Autodesk Fusion 360 part; units mm, degrees
note: some values were not read from the file. Chosen so that the rebuilt part matches the saved one: which bodies a step acts on. Set by a fixed rule: which sketch regions a step uses.
(part 2 of 2)
  constraint parallel L180 L182
  constraint parallel L181 L183
  constraint coincident L184 P96
  constraint coincident L185 P96
  constraint coincident P96 P95
  constraint horizontal L186
  constraint perpendicular L186 L187
  constraint parallel L186 L188
  constraint parallel L187 L189
  constraint coincident L190 P96
  constraint coincident L191 P96
  constraint horizontal L628
  constraint perpendicular L309 L628
  constraint parallel L283 L628
  constraint parallel L224 L309
  constraint coincident origin L301
  constraint coincident origin L300
  constraint perpendicular L621 L636
  constraint horizontal L312
  constraint perpendicular L312 L346
  constraint parallel L270 L312
  constraint parallel L346 L352
  constraint coincident P54 L298
  constraint coincident P54 L297
  constraint symmetric P54 P59 L621
  constraint symmetric L9.start L19.start L621
  constraint symmetric L15.end L19.end L621
  constraint symmetric L14.end L20.start L621
  constraint symmetric L9.end L21.end L621
  constraint symmetric L10.start L22.start L621
  constraint symmetric L10.end L22.end L621
  constraint symmetric L23.start L11.end L621
  constraint symmetric L12.end L23.end L621
  constraint horizontal L272
  constraint perpendicular L272 L349
  constraint parallel L272 L364
  constraint parallel L335 L349
  constraint coincident P57 L319
  constraint coincident P57 L269
  constraint vertical L234
  constraint symmetric P57 P61 L234
  constraint symmetric L31.start L40.start L234
  constraint symmetric L41.start L30.end L234
  constraint symmetric L32.end L42.end L234
  constraint symmetric L40.end L29.end L234
  constraint symmetric L42.start L32.start L234
  constraint symmetric L29.start L43.end L234
  constraint symmetric L45.start L36.end L234
  constraint symmetric L33.start L44.start L234
  constraint symmetric P57 P63 L621
  constraint symmetric L31.start L55.end L621
  constraint symmetric L50.end L30.end L621
  constraint symmetric L32.end L63.end L621
  constraint symmetric L29.end L50.start L621
  constraint symmetric L32.start L60.end L621
  constraint symmetric L51.start L29.start L621
  constraint symmetric L36.end L56.start L621
  constraint symmetric L56.end L33.start L621
  constraint symmetric L41.start L54.end L621
  constraint symmetric L44.start L52.end L621
  constraint symmetric L40.start L57.start L621
  constraint symmetric P61 P64 L621
  constraint symmetric L42.start L61.start L621
  constraint symmetric L45.start L52.start L621
  constraint symmetric L53.start L43.end L621
  constraint symmetric L42.end L58.start L621
  constraint symmetric L53.end L40.end L621
  constraint symmetric P64 P61 L621
  constraint coincident P66 L311
  constraint coincident P66 L316
  constraint perpendicular L271 L277
  constraint symmetric P66 P70 L277
  constraint symmetric L72.start L80.start L277
  constraint symmetric L74.end L78.end L277
  constraint symmetric L71.start L81.start L277
  constraint symmetric L72.end L80.end L277
  constraint symmetric L73.start L77.end L277
  constraint symmetric L74.start L78.start L277
  constraint symmetric L70.start L79.start L277
  constraint symmetric L70.end L77.start L277
  constraint symmetric P66 P71 L234
  constraint symmetric L72.start L84.start L234
  constraint symmetric L74.end L83.end L234
  constraint symmetric L71.start L87.end L234
  constraint symmetric L72.end L84.end L234
  constraint symmetric L73.start L87.start L234
  constraint symmetric L74.start L83.start L234
  constraint symmetric L70.start L86.start L234
  constraint symmetric L70.end L86.end L234
  constraint symmetric L76.start L95.start L234
  constraint symmetric L76.end L95.end L234
  constraint symmetric L78.end L94.end L234
  constraint symmetric P70 P72 L234
  constraint symmetric L89.start L77.start L234
  constraint symmetric L81.start L85.start L234
  constraint symmetric L79.start L85.end L234
  constraint symmetric L94.start L78.start L234
  constraint symmetric P72 P70 L234
  constraint symmetric L93.end L80.end L234
  constraint symmetric L89.end L77.end L234
  constraint symmetric L80.start L93.start L234
  constraint symmetric P47 L39.end L621
  constraint symmetric P44 P66 L621
  constraint symmetric L103.start L72.start L621
  constraint symmetric L109.end L74.end L621
  constraint symmetric L107.start L71.start L621
  constraint symmetric L103.end L72.end L621
  constraint symmetric L112.end L73.start L621
  constraint symmetric L109.start L74.start L621
  constraint symmetric L107.end L70.start L621
  constraint symmetric L70.end L110.end L621
  constraint symmetric L111.end L78.end L621
  constraint symmetric P45 P70 L621
  constraint symmetric L105.end L77.start L621
  constraint symmetric L96.end L81.start L621
  constraint symmetric L105.start L79.start L621
  constraint symmetric L111.start L78.start L621
  constraint symmetric L108.end L80.end L621
  constraint symmetric L96.start L77.end L621
  constraint symmetric L108.start L80.start L621
  constraint symmetric L115.end L84.end L621
  constraint symmetric L99.end L86.end L621
  constraint symmetric L98.end L85.start L621
  constraint symmetric L102.start L93.start L621
  constraint symmetric P46 P71 L621
  constraint symmetric L115.start L84.start L621
  constraint symmetric P43 P72 L621
  constraint symmetric L104.end L94.end L621
  constraint symmetric L114.start L83.start L621
  constraint symmetric L98.start L89.end L621
  constraint symmetric L87.start L106.end L621
  constraint symmetric L97.end L89.start L621
  constraint symmetric L117.end L87.end L621
  constraint symmetric L97.start L85.end L621
  constraint symmetric L94.start L104.start L621
  constraint symmetric L93.end L102.end L621
  constraint symmetric L99.start L86.start L621
  constraint symmetric L114.end L83.end L621
  constraint midpoint L120.start L221
  constraint parallel L213 L221
  constraint parallel L192 L221
  constraint parallel L216 L222
  constraint midpoint L125.start L278
  constraint perpendicular L246 L382
  constraint perpendicular L246 L376
  constraint midpoint P48 L355
  constraint midpoint L127.start L265
  constraint midpoint P39 L289
  constraint coincident L129.end L289
  constraint parallel L264 L273
  constraint symmetric L125.end L131.start L234
  constraint symmetric L126.end L130.start L234
  constraint symmetric L129.end L131.end L234
  constraint symmetric L125.end L133.start L621
  constraint symmetric L126.end L132.start L621
  constraint symmetric L129.end L133.end L621
  constraint symmetric L130.start L134.start L621
  constraint symmetric L131.start L135.start L621
  constraint symmetric L131.end L135.end L621
  constraint midpoint P49 L330
  constraint midpoint P50 L365
  constraint midpoint L136.start L357
  constraint midpoint P51 L279
  constraint midpoint P52 L274
  constraint parallel L330 L336
  constraint parallel L306 L330
  constraint coincident L140.end L357
  constraint coincident L141.end L279
  constraint parallel L337 L338
  constraint symmetric L138.end L143.start L277
  constraint symmetric L143.end L140.end L277
  constraint symmetric L141.end L142.end L277
  constraint symmetric L138.end L147.start L234
  constraint symmetric L140.end L147.end L234
  constraint symmetric L146.end L141.end L234
  constraint symmetric L145.end L142.end L234
  constraint symmetric L144.start L143.start L234
  constraint symmetric L143.end L144.end L234
  constraint symmetric L138.end L151.start L621
  constraint symmetric L140.end L151.end L621
  constraint symmetric L141.end L150.end L621
  constraint symmetric L142.end L149.end L621
  constraint symmetric L143.start L148.start L621
  constraint symmetric L143.end L148.end L621
  constraint symmetric L144.start L155.start L621
  constraint symmetric L144.end L155.end L621
  constraint symmetric L145.end L154.end L621
  constraint symmetric L146.end L153.end L621
  constraint symmetric L147.start L152.start L621
  constraint symmetric L152.end L147.end L621
  constraint perpendicular L267 L356
  constraint coincident L621.start L331
  constraint coincident L621.start L194
  constraint tangent L331 A15
  constraint tangent L194 A15
  constraint tangent L331 A8
  constraint tangent A8 L356
  constraint tangent L194 A6
  constraint tangent A6 L304
  constraint tangent L356 A9
  constraint tangent L267 A9
  constraint tangent L267 A7
  constraint tangent A7 L304
  constraint coincident L170.start L356
  constraint coincident P96 L621
  constraint symmetric L159.start L163.start L621
  constraint symmetric L161.end L162.end L621
  constraint symmetric L159.end L163.end L621
  constraint symmetric L160.start L164.start L621
  constraint symmetric L161.start L162.start L621
  constraint midpoint L167.end L267
  constraint coincident L165.start L621
  constraint coincident L165.end A5
  constraint coincident L165.end L621
  constraint collinear L236 L243
  constraint parallel L218 L371
  constraint coincident L172.start L304
  constraint collinear L286 L304
  constraint coincident L173.start L286
  constraint collinear L286 L299
  constraint horizontal L632
  constraint perpendicular L320 L632
  constraint parallel L313 L632
  constraint parallel L223 L320
  constraint horizontal L215
  constraint perpendicular L215 L351
  constraint parallel L215 L268
  constraint parallel L201 L351
  constraint coincident P96 L205
  constraint coincident P96 L200
  constraint horizontal L203
  constraint perpendicular L203 L322
  constraint parallel L203 L317
  constraint parallel L198 L322
  constraint coincident P96 L197
  constraint coincident P96 L195
  constraint horizontal L395
  constraint perpendicular L387 L395
  constraint parallel L388 L395
  constraint parallel L387 L408
  constraint coincident P75 L401
  constraint coincident P75 L393
  constraint coincident P75 P74
  constraint horizontal L396
  constraint perpendicular L386 L396
  constraint parallel L389 L396
  constraint parallel L386 L409
  constraint coincident P75 L397
  constraint coincident P75 L390
  constraint perpendicular L394 L396
  constraint coincident L404.end A13
  constraint midpoint L405.end L386
  constraint parallel L405 L407
  constraint coincident L407.end L386
  constraint coincident L406.end A13
  constraint parallel L404 L406
  constraint symmetric L404.start L385.start L394
  constraint symmetric L404.end L385.end L394
  constraint symmetric L405.end L391.end L394
  constraint symmetric L407.end L398.end L394
  constraint symmetric L406.start L402.start L394
  constraint symmetric L406.end L403.end L394
  constraint concentric A12 A13
  constraint coincident L391.start A10
  constraint coincident L398.start A10
  constraint coincident A17.start A16
  constraint concentric A15 A19
  constraint concentric A16 A17
  constraint symmetric A17.start L411.end L621
  constraint symmetric A15.end L410.end L621
  constraint coincident L411 A17.end
  constraint concentric A17 A18
  constraint concentric A19 A20
  constraint coincident L410 A18.start
  constraint coincident A21 L412.end
  constraint parallel L159 L412
  constraint horizontal L430
  constraint perpendicular L419 L430
  constraint parallel L430 L432
  constraint parallel L419 L427
  constraint coincident P96 L416
  constraint coincident P96 L421
  constraint horizontal L434
  constraint perpendicular L414 L434
  constraint parallel L434 L435
  constraint parallel L413 L414
  constraint coincident P96 L424
  constraint coincident P96 L415
  constraint horizontal L431
  constraint perpendicular L422 L431
  constraint parallel L428 L431
  constraint parallel L422 L429
  constraint coincident P96 L420
  constraint coincident P96 L425
  constraint horizontal L433
  constraint perpendicular L418 L433
  constraint parallel L433 L436
  constraint parallel L418 L423
  constraint coincident P96 L426
  constraint coincident P96 L417
  constraint horizontal L454
  constraint perpendicular L443 L454
  constraint parallel L454 L456
  constraint parallel L443 L451
  constraint coincident P96 L440
  constraint coincident P96 L445
  constraint horizontal L458
  constraint perpendicular L438 L458
  constraint parallel L458 L459
  constraint parallel L437 L438
  constraint coincident P96 L448
  constraint coincident P96 L439
  constraint horizontal L455
  constraint perpendicular L446 L455
  constraint parallel L452 L455
  constraint parallel L446 L453
  constraint coincident P96 L444
  constraint coincident P96 L449
  constraint horizontal L457
  constraint perpendicular L442 L457
  constraint parallel L457 L460
  constraint parallel L442 L447
  constraint coincident P96 L450
  constraint coincident P96 L441
  constraint horizontal L478
  constraint perpendicular L467 L478
  constraint parallel L478 L480
  constraint parallel L467 L475
  constraint coincident P96 L464
  constraint coincident P96 L469
  constraint horizontal L482
  constraint perpendicular L462 L482
  constraint parallel L482 L483
  constraint parallel L461 L462
  constraint coincident P96 L472
  constraint coincident P96 L463
  constraint horizontal L479
  constraint perpendicular L470 L479
  constraint parallel L476 L479
  constraint parallel L470 L477
  constraint coincident P96 L468
  constraint coincident P96 L473
  constraint horizontal L481
  constraint perpendicular L466 L481
  constraint parallel L481 L484
  constraint parallel L466 L471
  constraint coincident P96 L474
  constraint coincident P96 L465
  constraint coincident A21 L493.end
  constraint parallel L199 L493
  constraint coincident A21 L494.end
  constraint perpendicular L496 L497
  constraint parallel L496 L500
  constraint perpendicular L514 L515
  constraint parallel L513 L515
  constraint parallel L514 L517
  constraint symmetric L39 L513.end L520.start
  constraint symmetric L39 L515.start L520.end
  constraint symmetric L39 L511.start L521.end
  constraint symmetric L39 L511.end L524.end
  constraint symmetric L39 L513.start L523.end
  constraint symmetric L39 L514.start L522.end
  constraint symmetric L39 L516.start L519.end
  constraint symmetric L39 L512.end L519.start
  constraint symmetric L277 L543.end L547.end
  constraint symmetric L277 L543.start L547.start
  constraint symmetric L277 L545.end L549.start
  constraint symmetric L277 L544.start L548.start
  constraint symmetric L39 L543.end L551.end
  constraint symmetric L39 L543.start L551.start
  constraint symmetric L39 L545.end L553.start
  constraint symmetric L39 L544.start L552.start
  constraint symmetric L39 L547.start L555.start
  constraint symmetric L39 L547.end L555.end
  constraint symmetric L39 L548.start L556.start
  constraint symmetric L39 L549.start L557.end
  constraint coincident L508 L123.start
  constraint coincident L508 L122.start
  constraint coincident L498 L124.start
  constraint coincident L498 L307.start
  constraint coincident L485 L124.end
  constraint coincident L485 L307.end
  constraint coincident L486 L123.end
  constraint coincident L486 L122.end
  constraint coincident L492 L405.start
  constraint coincident L499 L128.end
  constraint coincident L501 L130.end
  constraint coincident L543 L142.start
  constraint coincident L547 L141.start
  constraint coincident L555 L146.start
  constraint coincident L551 L145.start
  constraint coincident L573 L154.start
  constraint coincident L569 L153.start
  constraint coincident L566 L150.start
  constraint coincident L560 L149.start
  constraint perpendicular L577 L581
  constraint parallel L577 L582
  constraint parallel L578 L581
  constraint perpendicular L580 L583
  constraint parallel L576 L583
  constraint parallel L579 L580
  constraint coincident A13 A22.start
  constraint coincident A12 A22.end
  constraint symmetric L394 A13.start A13.end
  constraint symmetric L394 A22.start A25.end
  constraint symmetric L394 A22 A25
  constraint symmetric L394 A23 A24
  constraint symmetric L394 A22.end A25.start
  constraint symmetric L394 A12.end A12.start
  constraint tangent A15 S0
  constraint tangent A19 S1
  constraint concentric A30 A31
  constraint coincident A31.end S0
  constraint coincident A31.start S1
  constraint midpoint A30.end L584
  constraint midpoint A30.start L585
  constraint tangent A19 S2
  constraint tangent A18 S3
  constraint coincident A32 S2.end
  constraint midpoint S2.end L588
  constraint coincident A32 S3.start
  constraint midpoint S3.start L589
  constraint coincident A32 L586.end
  constraint coincident A32 L587.end
  constraint concentric A33 A34
  constraint concentric A35 A36
  constraint coincident A34.start S5
  constraint coincident A34.end S6
  constraint coincident A35.end S6
  constraint coincident A35.start S4
  constraint midpoint A36.start L590
  constraint midpoint A33.start L591
  constraint midpoint A33.end L592
  constraint midpoint A36.end L593
  constraint midpoint A37.end L594
  constraint collinear L595 L596
  constraint midpoint A37.start L597
  constraint midpoint A39.start L598
  constraint midpoint A39.end L599
  constraint concentric A41 A42
  constraint coincident A41.end L600
  constraint coincident A41.start L600
  constraint coincident A42.end L600
  constraint collinear L600 L601
  constraint symmetric L234 A41.end A43.start
  constraint symmetric L234 A41.start A43.end
  constraint symmetric L234 A41 A43
  constraint symmetric L234 A42.end A44.start
  constraint symmetric L234 A42.start A44.end
  constraint symmetric L234 A42 A44
  constraint concentric A45 A46
  constraint coincident A46.start L601
  constraint coincident A45.start L601
  constraint coincident A46.end L601
  constraint collinear L601 L602
  constraint collinear L602 L603
  constraint coincident L286 L605.end
  constraint perpendicular L286 L604
  constraint collinear L604 L606
  constraint collinear L605 L606
  constraint collinear L606 L607
  constraint symmetric A52.start L606 L606.start
  constraint symmetric L604.end L606 A52.end
  constraint symmetric A49.start L606 L606.end
  constraint symmetric L607.start L606 A49.end
  constraint symmetric L605.start L606 A47.start
  constraint symmetric L607.end L606 A47.end
  constraint coincident A53 S10.end
  constraint midpoint S10.end L608
  constraint coincident A53 S11.start
  constraint midpoint S11.start L609
  constraint coincident A54 S12.end
  constraint midpoint S12.end L610
  constraint coincident A54 S13.start
  constraint midpoint S13.start L611
  constraint coincident S11 A55.end
  constraint coincident S10 A56.start
  constraint concentric A55 A56
  constraint tangent A2 L612
  constraint collinear L612 L613
  constraint coincident A58 L613.end
  constraint coincident A58 L614.start
  constraint collinear L613 L614
  constraint parallel L167 L619
  constraint symmetric L39 A58 A59
  constraint tangent A60 L615
  constraint tangent A60 L616
  constraint collinear L618 L621
  constraint coincident L615 L619.end
  constraint coincident L616 L620.start
  constraint collinear L619 L620
  constraint concentric A59 A60
  constraint coincident A65 L621.end
  constraint coincident A65 L624.start
  constraint collinear L621 L624
  constraint coincident A65 L622.end
  constraint coincident A65 L623.start
  constraint collinear L622 L623
  constraint coincident A61 L624.end
  constraint coincident A61 L625.start
  constraint collinear L624 L625
  constraint coincident A61 L166.start
  constraint coincident A61 L623.end
  constraint coincident L491 L626.end
  constraint collinear L626 L627
  constraint coincident L489 L627.start
  constraint collinear L628 L629
  constraint collinear L630 L631
  constraint collinear L632 L633
  constraint coincident L491 L634.end
  constraint coincident L621 L635.start
  constraint collinear L634 L635
  constraint collinear L636 L637
  constraint tangent A58 S14
  constraint tangent A58 S15
  measures "d1" distance of L0.end L1.end
  measures "d2" distance of L0.start L0.end
  measures "d4" distance of L6.end L7.end
  measures "d6" distance of L15.end L9.end
  measures "d7" distance of L9.start L15.end
  measures "d8" distance of L10.start L12.end
  measures "d10" distance of L30.end L29.end
  measures "d11" distance of L29.end L29.start
  measures "d12" distance of L32.end L32.start
  measures "d14" distance of L74.end L72.end
  measures "d15" distance of L72.end L74.start
  measures "d16" distance of L71.start L73.start
  measures "d20" distance of L120.start L120.end
  measures "d21" distance of L120.start L121.end
  measures "d22" angle of L26 L122
  measures "d23" distance of L125.start L125.end L44.start
  measures "d24" distance of L125.start L126.end L44.start
  measures "d27" distance of P49 L138.end
  measures "d28" distance of P49 L139.end
  measures "d30" distance of L86 L156
  measures "d31" radius of A16
  measures "d32" radius of A0
  measures "d34" radius of A2
  measures "d36" diameter of A4
  measures "d90" distance of L0.end L1.end
  measures "d91" distance of L0.start L0.end
  measures "d92" distance of L7.end L6.end
  measures "d93" distance of L181.end L182.end
  measures "d94" distance of L180.end L181.end
  measures "d95" distance of L187.end L188.end
  measures "d96" distance of L186.end L187.end
  measures "d107" distance of L0.end L1.end
  measures "d108" distance of L0.start L0.end
  measures "d109" distance of L7.end L6.end
  measures "d110" distance of L15.end L9.end
  measures "d111" distance of L9.start L15.end
  measures "d112" distance of L10.start L12.end
  measures "d113" distance of L30.end L29.end
  measures "d114" distance of L29.start L29.end
  measures "d115" distance of L32.end L32.start
  measures "d116" distance of L74.end L72.end
  measures "d117" distance of L72.end L74.start
  measures "d118" distance of L71.start L73.start
  measures "d119" distance of L120.start L120.end
  measures "d120" distance of L120.start L121.end
  measures "d121" angle of L221 L222
  measures "d122" distance of L125.end L125.start
  measures "d123" distance of L126.end L125.start
  measures "d124" distance of L138.end P49
  measures "d125" distance of P49 L139.end
  measures "d126" distance of L267 L360
  measures "d127" radius of A15
  measures "d128" radius of A8
  measures "d129" radius of A9
  measures "d130" diameter of A5
  measures "d147" distance of L1.end L0.end
  measures "d148" distance of L0.start L0.end
  measures "d149" distance of L7.end L6.end
  measures "d150" distance of L182.end L181.end
  measures "d151" distance of L180.end L181.end
  measures "d152" distance of L187.end L188.end
  measures "d153" distance of L187.end L186.end
  measures "d164" diameter of A13
  measures "d165" distance of L387.end L388.end
  measures "d166" distance of L387.end L387.start
  measures "d167" distance of L389.end L386.end
  measures "d168" distance of L386.end L386.start
  measures "d191" distance of L182.end L181.end
  measures "d192" distance of L181.end L180.end
  measures "d193" distance of L188.end L187.end
  measures "d194" distance of L186.end L187.end
  measures "d195" distance of L181.end L182.end
  measures "d196" distance of L181.end L180.end
  measures "d197" distance of L187.end L188.end
  measures "d198" distance of L187.end L186.end
  measures "d199" distance of L182.end L181.end
  measures "d200" distance of L181.end L180.end
  measures "d201" distance of L188.end L187.end
  measures "d202" distance of L186.end L187.end
  measures "d203" distance of L181.end L182.end
  measures "d204" distance of L181.end L180.end
  measures "d205" distance of L187.end L188.end
  measures "d206" distance of L187.end L186.end
  measures "d207" distance of L182.end L181.end
  measures "d208" distance of L181.end L180.end
  measures "d209" distance of L188.end L187.end
  measures "d210" distance of L186.end L187.end
  measures "d211" distance of L181.end L182.end
  measures "d212" distance of L181.end L180.end
  measures "d213" distance of L187.end L188.end
  measures "d214" distance of L187.end L186.end
  measures "d215" distance of L489.start L488.start
  measures "d216" distance of L490.start L486.end
  measures "d217" distance of L487.start L488.start
  measures "d218" distance of L500.start L496.end
  measures "d219" distance of L496.end L496.start
  measures "d220" distance of L498.start L495.start
  measures "d221" distance of L496.end L500.start
  measures "d222" distance of L513.end L513.start
  measures "d223" distance of L513.start L514.start
  measures "d224" distance of L511.start L516.start
  measures "d226" distance of L543.end L543.start
  measures "d300" distance of L578.start L581.end
  measures "d301" distance of L581.end L577.end
  measures "d302" distance of L576.start L576.end
  measures "d303" distance of L576.start L580.start
  measures "d376" radius of A58
  measures "d377" radius of A57
extrude "Extrusão73" add sketch "Esboço1" along normal blind 4 contours L7 L8 L158 L161 L179 L266 L307 L314 L315 L321 L331 A18 A20 L485 L490 L559 A32 L587 S3 L589 A33 S5 L591 S6 L592 L635 L637 | L405 A17 A19 L490 L492 A31 S1 A32 L586 S2 | L5 L8 L124 A4 L159 L160 L174 L179 A5 L214 L233 L308 L314 L318 L321 L345 L485 A35 S4 S6 L593 | L5 L6 L122 A4 L163 L164 L174 L175 A5 L199 L214 L217 L222 L225 L228 L233 L486 A38 S7 S8 L597 | L6 L7 L123 L157 L162 L175 L194 L216 L225 L227 L228 L266 L407 A15 A16 L486 L492 A31 S0 A39 S8 L598 S9 L599 L634 L636 makes body 1 at (50.6885, -2.7666, 4) makes body 2 at (-4.4582, 27.7889, 4) makes body 3 at (41.1604, -31.7588, 0) makes body 4 at (-50.6869, -2.7681, 0) makes body 5 at (-41.1604, -31.7588, 0)
extrude "Extrusão74" add sketch "Esboço1" along normal blind 2 contours L0 L178 L309 L320 L490 L627 L629 L631 L633 | L0 L7 L8 L178 L179 L266 L309 L314 L320 L321 L490 L627 L629 L631 L633 L635 L637 | L0 L178 L309 L320 L489 L490 L627 L629 L631 L633 | L0 L8 L178 L179 L309 L314 L320 L321 L489 L490 | L7 L266 L489 L490 L627 L629 L631 L633 L635 L637 | L0 L1 L2 L7 L176 L177 L178 L223 L224 L266 L283 L309 L313 L320 L487 L488 L489 L491 L635 L637 | L0 L8 L178 L179 L309 L314 L320 L321 L488 L489 | L8 L179 L314 L321 L485 L488 L489 L490 | L7 L266 L489 L490 L491 L492 L634 L635 L636 L637 | L0 L1 L177 L178 L283 L309 L313 L320 L485 L488 | L0 L8 L178 L179 L309 L314 L320 L321 L485 L488 | L8 L179 L314 L321 L488 L489 | L7 L266 L489 L491 L635 L637 | L0 L1 L177 L178 L283 L309 L313 L320 L485 | L0 L1 L5 L8 L174 L177 L178 L179 L214 L233 L283 L309 L313 L314 L320 L321 L485 | L1 L5 L174 L177 L214 L233 L283 L313 L485 L488 | L1 L5 L174 L177 L214 L233 L283 L313 L487 L488 | L1 L2 L176 L177 L223 L224 L283 L313 L486 L487 | L1 L5 L174 L177 L214 L233 L283 L313 L486 L487 | L5 A4 L174 A5 L214 L233 L485 L486 L487 L488 | L5 L174 L214 L233 L487 L488 | L7 L266 L491 L492 L626 L628 L630 L632 L634 L636 | L1 L2 L176 L177 L223 L224 L283 L313 L486 | L1 L2 L5 L6 L174 L175 L176 L177 L214 L223 L224 L225 L228 L233 L283 L313 L486 | L2 L6 L175 L176 L223 L224 L225 L228 L486 L487 | L2 L6 L175 L176 L223 L224 L225 L228 L487 L491 | L2 L6 L7 L175 L176 L223 L224 L225 L228 L266 L492 L626 L628 L630 L632 L634 L636 | L2 L176 L223 L224 L491 L492 L626 L628 L630 L632 | A4 A5 A21 L412 L485 L486 L493 | L2 L6 L175 L176 L223 L224 L225 L228 L491 L492 | L6 L175 L225 L228 L486 L487 L491 L492 | L6 L175 L225 L228 L487 L491 | L2 L176 L223 L224 L492 L626 L628 L630 L632 bodies 1 5 2 3 4
extrude "Extrusão75" add sketch "Esboço1" along normal blind 6 contours L7 L266 L490 A32 L586 L587 L635 L637 | L124 L307 L308 L485 L559 S6 | L7 L266 L405 L407 L492 A31 L634 L636 | L122 L123 L216 L222 L486 S8 bodies 1
extrude "Extrusão76" add sketch "Esboço1" along normal blind 4 separate body contours L10 L11 L13 L32 L36 L37 L131 L143 L158 A0 L161 L170 L171 L265 L271 L281 L307 L310 L315 L323 L329 L331 L339 A8 L350 L356 L357 L495 L498 L501 L511 L512 L516 L559 A34 S5 S6 L592 A42 L600 L601 A57 L612 L613 | L11 L12 L13 L42 L45 L47 L124 L129 L144 A4 L159 L160 L165 L166 A5 L229 L243 L264 L265 L278 L308 L310 L318 L340 L344 L345 L354 L355 L498 L499 L521 L524 L525 A36 S4 L590 S6 L593 A44 L602 L603 L604 A62 A64 A65 L622 L623 | L32 L33 L37 L42 L44 L45 L128 L130 L140 L147 L271 L273 L278 L280 L334 L338 L340 L342 L353 L357 L499 L501 L516 L518 L519 L521 A46 L601 L602 | L145 L146 L325 L348 L519 L525 L602 | L141 L142 L333 L337 L512 L518 L601 makes body 6 at (-61.0053, -127.9109, 0) makes body 7 at (-100, -146.0948, 0) makes body 8 at (-148.8162, -124.6972, 0) makes body 9 at (-150, -213.7, 0) makes body 10 at (-50, -213.7, 0)
extrude "Extrusão77" add sketch "Esboço1" along normal blind 6 contours L124 L307 L308 L498 L559 S6 | L11 L128 L129 L264 L265 L273 L499 L521 | L11 L130 L131 L265 L280 L281 L501 L516 | L45 L144 L145 L340 L348 L354 L525 L602 | L37 L142 L143 L333 L350 L357 L512 L601 | L45 L146 L147 L325 L340 L353 L519 L602 | L37 L140 L141 L337 L338 L357 L518 L601 bodies 6 7 8
extrude "Extrusão78" add sketch "Esboço1" along normal blind 2 contours L13 L310 L495 L496 L497 L498 | A4 A5 A21 L412 L494 | L13 L17 L310 L312 L497 L498 | L12 L13 L14 L17 L310 L312 L352 L355 L498 | L10 L13 L17 L18 L310 L312 L329 L346 L495 | L13 L17 L310 L312 L495 L496 | L13 L17 L310 L312 L496 L497 | L13 L310 L496 L497 | L14 L17 L312 L352 L497 L498 | L14 L17 L312 L352 L498 | L17 L18 L312 L346 L495 | L17 L18 L312 L346 L495 L496 | L12 L355 L497 L498 L499 L500 | L12 L14 L352 L355 L497 L498 | L14 L16 L17 L18 L270 L312 L346 L352 L496 L497 L500 L502 | L10 L18 L329 L346 L495 L496 | L10 L329 L495 L496 L501 L502 | L12 L355 L497 L500 | L12 L14 L352 L355 L497 L500 | L10 L18 L329 L346 L496 L502 | L10 L329 L496 L502 | L12 L14 L352 L355 L499 L500 | L11 L12 L14 L16 L265 L270 L352 L355 L499 | L14 L16 L270 L352 L499 L500 | L16 L18 L270 L346 L501 L502 | L10 L18 L329 L346 L501 L502 | L10 L11 L16 L18 L265 L270 L329 L346 L501 | L14 L16 L270 L352 L499 | L11 L16 L265 L270 L500 L502 | L11 L16 L265 L270 L499 L500 | L16 L18 L270 L346 L501 | L11 L16 L265 L270 L501 L502 | L11 L265 L500 L502 | L11 L265 L499 L500 L501 L502 | L42 L129 L264 L278 L521 L522 L523 L524 | L128 L129 L264 L273 L521 L522 | L130 L131 L280 L281 L515 L516 | L32 L131 L271 L281 L511 L514 L515 L516 | L42 L129 L264 L278 L522 L523 | L42 L128 L129 L264 L273 L278 L522 | L42 L128 L273 L278 L521 L522 | L32 L130 L131 L271 L280 L281 L515 | L32 L131 L271 L281 L514 L515 | L32 L130 L271 L280 L515 L516 | L42 L43 L278 L282 L522 L523 | L42 L128 L273 L278 L522 | L41 L42 L43 L44 L278 L282 L327 L334 L521 | L42 L43 L278 L282 L521 L522 | L42 L43 L278 L282 L523 L524 | L42 L43 L47 L49 L278 L282 L343 L344 L524 | L32 L38 L271 L272 L514 L515 | L32 L130 L271 L280 L515 | L32 L38 L271 L272 L515 L516 | L32 L33 L34 L38 L271 L272 L335 L342 L516 | L29 L32 L36 L38 L271 L272 L323 L349 L511 | L32 L38 L271 L272 L511 L514 | L41 L43 L282 L327 L521 | L41 L43 L282 L327 L521 L522 | L43 L49 L282 L343 L523 L524 | L43 L49 L282 L343 L524 | L34 L38 L272 L335 L515 L516 | L34 L38 L272 L335 L516 | L29 L38 L272 L349 L511 | L29 L38 L272 L349 L511 L514 | L41 L43 L46 L49 L282 L324 L327 L343 L520 L522 L523 L526 | L41 L44 L327 L334 L521 L522 | L44 L334 L519 L520 L521 L522 | L47 L344 L523 L524 L525 L526 | L47 L49 L343 L344 L523 L524 | L29 L30 L34 L38 L272 L335 L349 L364 L513 L514 L515 L517 | L33 L342 L515 L516 L517 L518 | L33 L34 L335 L342 L515 L516 | L29 L36 L323 L349 L511 L514 | L36 L323 L511 L512 L513 L514 | L45 L46 L47 L49 L324 L340 L343 L344 L525 | L47 L49 L343 L344 L523 L526 | L41 L44 L327 L334 L520 L522 | L44 L334 L520 L522 | L47 L344 L523 L526 | L29 L36 L323 L349 L513 L514 | L33 L34 L335 L342 L515 L517 | L33 L342 L515 L517 | L36 L323 L513 L514 | L29 L30 L36 L37 L323 L349 L357 L364 L512 | L45 L46 L324 L340 L525 L526 | L45 L145 L146 L325 L340 L348 L519 L520 L525 L526 | L47 L49 L343 L344 L525 L526 | L46 L49 L324 L343 L525 L526 | L41 L46 L324 L327 L519 L520 | L41 L44 L327 L334 L519 L520 | L41 L44 L45 L46 L324 L327 L334 L340 L519 | L29 L30 L349 L364 L512 L513 | L29 L36 L323 L349 L512 L513 | L33 L34 L335 L342 L517 L518 | L30 L34 L335 L364 L517 L518 | L30 L33 L34 L37 L335 L342 L357 L364 L518 | L30 L37 L357 L364 L512 L513 | L37 L142 L333 L357 L512 | L37 L141 L142 L333 L337 L357 L512 L513 L517 L518 | L46 L49 L324 L343 L525 | L45 L46 L324 L340 L520 L526 | L41 L46 L324 L327 L519 | L45 L46 L324 L340 L519 L520 | L29 L30 L349 L364 L512 | L30 L37 L357 L364 L513 L517 | L30 L34 L335 L364 L518 | L30 L37 L357 L364 L517 L518 | L37 L141 L337 L357 L518 | L45 L340 L520 L526 | L37 L357 L513 L517 bodies 6 9 10
extrude "Extrusão79" add sketch "Esboço1" along normal blind 4 separate body contours L23 L24 L26 L52 L58 L61 L122 L133 L155 A4 L163 L164 L165 L166 A5 L196 L199 L208 L217 L219 L220 L221 L222 L229 L243 L245 L251 L255 L506 L508 L537 L540 L542 A37 S7 L594 S8 L597 L604 L606 A51 A61 A63 A66 L622 L623 | L22 L24 L26 L56 L63 L65 L123 L135 L148 L157 A1 L162 L172 L173 L194 L202 L207 L209 L216 L220 L221 L227 A6 L258 L286 L293 L299 L303 L504 L508 L510 L527 L530 L534 A40 S8 L598 S9 L605 L607 A48 A53 S10 L608 S11 L609 | L153 L154 L252 L253 L535 L542 L606 | L52 L56 L60 L61 L63 L67 L132 L134 L151 L152 L206 L209 L210 L219 L245 L248 L260 L263 L293 L302 L504 L506 L532 L534 L535 L537 L606 L607 A49 | L149 L150 L284 L285 L530 L532 L607 makes body 11 at (148.8208, -124.6973, 0) makes body 12 at (100, -146.0948, 0) makes body 13 at (150, -213.7, 0) makes body 14 at (61.0053, -127.9109, 0) makes body 15 at (50, -213.7, 0)
extrude "Extrusão80" add sketch "Esboço1" along normal blind 6 contours L122 L123 L216 L222 L508 S8 | L52 L154 L155 L245 L251 L253 L542 L606 | L24 L132 L133 L208 L210 L220 L506 L537 | L52 L152 L153 L245 L248 L252 L535 L606 | L24 L134 L135 L206 L207 L220 L504 L534 | L56 L150 L151 L285 L293 L302 L532 L607 | L56 L148 L149 L284 L293 L303 L530 L607 bodies 11 12 13 14 15
extrude "Extrusão81" add sketch "Esboço1" along normal blind 2 contours A4 A5 A21 L493 L494 | L26 L221 L507 L508 L509 L510 | L20 L23 L25 L26 L196 L204 L221 L232 L508 | L20 L26 L221 L232 L507 L508 | L26 L221 L507 L509 | L20 L26 L221 L232 L507 L509 | L20 L25 L204 L232 L508 | L20 L25 L204 L232 L507 L508 | L20 L26 L221 L232 L509 L510 | L19 L20 L22 L26 L193 L202 L221 L232 L510 | L23 L25 L196 L204 L507 L508 | L23 L196 L505 L506 L507 L508 | L19 L20 L25 L27 L193 L204 L212 L232 L503 L505 L507 L509 | L19 L20 L193 L232 L509 L510 | L19 L20 L193 L232 L510 | L23 L25 L196 L204 L505 L507 | L23 L196 L505 L507 | L22 L202 L503 L504 L509 L510 | L19 L22 L193 L202 L509 L510 | L23 L25 L196 L204 L505 L506 | L23 L24 L25 L27 L196 L204 L212 L220 L506 | L19 L22 L193 L202 L503 L509 | L25 L27 L204 L212 L505 L506 | L22 L202 L503 L509 | L25 L27 L204 L212 L506 | L19 L22 L193 L202 L503 L504 | L19 L27 L193 L212 L503 L504 | L24 L27 L212 L220 L505 L506 | L24 L27 L212 L220 L503 L505 | L19 L22 L24 L27 L193 L202 L212 L220 L504 | L19 L27 L193 L212 L504 | L24 L27 L212 L220 L503 L504 | L24 L132 L134 L206 L210 L220 L503 L504 L505 L506 | L24 L220 L503 L505 | L52 L53 L58 L69 L245 L255 L256 L384 L542 | L24 L132 L210 L220 L506 | L132 L133 L208 L210 L537 L538 | L61 L133 L208 L219 L537 L538 L539 L540 | L52 L69 L245 L384 L541 L542 | L52 L154 L245 L253 L542 | L52 L153 L154 L245 L252 L253 L535 L536 L541 L542 | L61 L132 L133 L208 L210 L219 L538 | L61 L133 L208 L219 L538 L539 | L61 L132 L210 L219 L537 L538 | L24 L134 L206 L220 L504 | L58 L255 L539 L540 L541 L542 | L53 L58 L255 L256 L541 L542 | L53 L69 L256 L384 L541 L542 | L53 L69 L256 L384 L542 | L52 L153 L245 L252 L535 | L63 L135 L207 L209 L527 L528 L533 L534 | L134 L135 L206 L207 L533 L534 | L57 L61 L219 L226 L538 L539 | L61 L132 L210 L219 L538 | L57 L61 L219 L226 L537 L538 | L57 L61 L64 L67 L219 L226 L261 L263 L537 | L53 L57 L58 L61 L219 L226 L255 L256 L540 | L57 L61 L219 L226 L539 L540 | L58 L255 L539 L541 | L53 L58 L255 L256 L539 L541 | L52 L69 L245 L384 L536 L541 | L52 L245 L536 L541 | L53 L57 L64 L69 L226 L256 L261 L384 L536 L538 L539 L541 | L52 L69 L245 L384 L535 L536 | L52 L64 L67 L69 L245 L261 L263 L384 L535 | L63 L135 L207 L209 L528 L533 | L63 L134 L135 L206 L207 L209 L533 | L63 L134 L206 L209 L533 L534 | L57 L64 L226 L261 L537 L538 | L57 L64 L226 L261 L537 | L53 L57 L226 L256 L540 | L53 L57 L226 L256 L539 L540 | L53 L58 L255 L256 L539 L540 | L64 L69 L261 L384 L535 L536 | L64 L69 L261 L384 L535 | L63 L68 L209 L211 L528 L533 | L63 L134 L206 L209 L533 | L55 L60 L63 L68 L209 L211 L260 L262 L534 | L63 L68 L209 L211 L533 L534 | L63 L68 L209 L211 L527 L528 | L51 L63 L65 L68 L209 L211 L254 L258 L527 | L67 L263 L535 L536 L537 L538 | L64 L67 L261 L263 L537 L538 | L64 L67 L261 L263 L535 L536 | L64 L67 L261 L263 L536 L538 | L55 L68 L211 L262 L534 | L55 L68 L211 L262 L533 L534 | L51 L68 L211 L254 L527 L528 | L51 L68 L211 L254 L527 | L67 L263 L536 L538 | L50 L55 L56 L60 L260 L262 L292 L293 L532 | L50 L51 L55 L68 L211 L254 L262 L292 L528 L529 L531 L533 | L55 L60 L260 L262 L533 L534 | L60 L260 L531 L532 L533 L534 | L65 L258 L527 L528 L529 L530 | L51 L65 L254 L258 L527 L528 | L50 L56 L292 L293 L531 L532 | L56 L150 L285 L293 L532 | L56 L149 L150 L284 L285 L293 L529 L530 L531 L532 | L51 L65 L254 L258 L528 L529 | L55 L60 L260 L262 L531 L533 | L60 L260 L531 L533 | L65 L258 L528 L529 | L55 L60 L260 L262 L531 L532 | L50 L55 L262 L292 L531 L532 | L50 L55 L262 L292 L532 | L56 L149 L284 L293 L530 | L51 L65 L254 L258 L529 L530 | L50 L51 L254 L292 L529 L530 | L50 L51 L56 L65 L254 L258 L292 L293 L530 | L50 L56 L292 L293 L529 L531 | L56 L293 L529 L531 | L50 L56 L292 L293 L529 L530 | L50 L51 L254 L292 L530 bodies 11
extrude "Extrusão82" add sketch "Esboço1" along normal blind 4 separate body contours L70 L71 L73 L75 L77 L79 L81 L82 L85 L86 L87 L88 L89 L90 L91 L92 L140 L141 L142 L143 L144 L145 L146 L147 L156 A2 L166 L167 L170 L236 L243 L267 L325 L326 L328 L330 L333 L337 L338 L339 L341 L348 L350 L353 L354 L358 L359 L360 L361 L362 L363 L365 L366 L367 L368 L369 L370 A9 L543 L544 L545 L546 L547 L548 L549 L550 L551 L552 L553 L554 L555 L556 L557 L558 A41 L600 A43 A45 L601 L602 L603 L604 A58 L613 L614 A59 A60 L615 L616 L619 L620 S14 S15 makes body 16
extrude "Extrusão83" add sketch "Esboço1" along normal blind 6 contours L87 L144 L145 L348 L354 L367 L551 L602 | L73 L142 L143 L333 L350 L365 L543 L601 | L91 L146 L147 L325 L341 L353 L555 L602 | L82 L140 L141 L330 L337 L338 L547 L601 bodies 16
extrude "Extrusão84" add sketch "Esboço1" along normal blind 2 contours L87 L88 L367 L369 L551 | L71 L73 L362 L365 L543 | L86 L87 L88 L90 L360 L367 L368 L369 L551 L552 L553 L554 | L87 L367 L551 L552 | L73 L365 L543 L544 | L70 L71 L73 L75 L361 L362 L365 L370 L543 L544 L545 L546 | L88 L369 L551 L554 | L87 L90 L367 L368 L552 | L91 L341 L555 L556 | L71 L362 L543 L545 | L73 L75 L365 L370 L544 | L82 L330 L547 L548 | L86 L88 L360 L369 L554 | L90 L368 L552 L553 | L85 L91 L328 L341 L555 | L85 L89 L91 L92 L328 L341 L363 L366 L555 L556 L557 L558 | L70 L71 L361 L362 L545 | L75 L370 L544 L546 | L77 L79 L81 L82 L326 L330 L358 L359 L547 L548 L549 L550 | L81 L82 L330 L359 L547 | L86 L360 L553 L554 | L86 L90 L360 L368 L553 | L89 L91 L341 L363 L556 | L85 L328 L555 L557 | L70 L361 L545 L546 | L70 L75 L361 L370 L546 | L77 L82 L330 L358 L548 | L81 L359 L547 L550 | L89 L363 L556 L558 | L85 L92 L328 L366 L557 | L77 L358 L548 L549 | L79 L81 L326 L359 L550 | L89 L92 L363 L366 L558 | L92 L366 L557 L558 | L77 L79 L326 L358 L549 | L79 L326 L549 L550 bodies 16
extrude "Extrusão85" add sketch "Esboço1" along normal blind 4 separate body contours L96 L97 L98 L99 L100 L101 L105 L106 L107 L110 L112 L113 L116 L117 L118 L119 L148 L149 L150 L151 L152 L153 L154 L155 L156 A3 L166 L167 L169 L172 L235 L236 L238 L240 L243 L244 L248 L250 L251 L252 L253 L257 L259 L267 A7 L284 L285 L286 L287 L288 L290 L291 L296 L302 L303 L304 L305 L371 L377 L378 L560 L561 L562 L563 L564 L565 L566 L567 L568 L569 L570 L571 L572 L573 L574 L575 L604 L605 L606 L607 A47 A50 A52 A54 S12 L610 S13 L611 A59 A60 L615 L616 L619 L620 makes body 17
extrude "Extrusão86" add sketch "Esboço1" along normal blind 6 contours L117 L154 L155 L235 L251 L253 L573 L606 | L98 L152 L153 L248 L252 L259 L569 L606 | L96 L150 L151 L285 L302 L378 L566 L607 | L118 L148 L149 L284 L288 L303 L560 L607 bodies 17
extrude "Extrusão87" add sketch "Esboço1" along normal blind 2 contours L117 L119 L235 L250 L573 | L117 L235 L572 L573 | L99 L106 L117 L119 L235 L240 L244 L250 L572 L573 L574 L575 | L119 L250 L573 L574 | L106 L117 L235 L244 L572 | L98 L259 L569 L570 | L99 L119 L240 L250 L574 | L106 L244 L572 L575 | L97 L98 L100 L101 L238 L257 L259 L371 L568 L569 L570 L571 | L98 L100 L259 L371 L569 | L99 L240 L574 L575 | L99 L106 L240 L244 L575 | L98 L101 L238 L259 L570 | L100 L371 L568 L569 | L101 L238 L570 L571 | L97 L100 L257 L371 L568 | L97 L101 L238 L257 L571 | L97 L257 L568 L571 | L96 L116 L296 L378 L566 | L96 L378 L564 L566 | L96 L105 L113 L116 L290 L296 L377 L378 L564 L565 L566 L567 | L116 L296 L566 L567 | L96 L113 L290 L378 L564 | L118 L288 L560 L561 | L107 L118 L288 L291 L560 | L105 L116 L296 L377 L567 | L113 L290 L564 L565 | L107 L110 L112 L118 L287 L288 L291 L305 L560 L561 L562 L563 | L105 L377 L565 L567 | L105 L113 L290 L377 L565 | L112 L118 L288 L305 L561 | L107 L291 L560 L562 | L112 L305 L561 L563 | L107 L110 L287 L291 L562 | L110 L112 L287 L305 L563 | L110 L287 L562 L563 bodies 17
extrude "Extrusão88" add sketch "Esboço1" along normal blind 4 separate body contours L386 L389 L391 A12 L405 L409 L576 L579 L580 L583 A22 A25 A27 A28 | L386 L396 L398 A13 L407 L409 L579 L583 A22 A25 A27 A28 makes body 18 at (186.0597, 65.4831, 0) makes body 19 at (234.5401, 114.606, 0)
extrude "Extrusão89" add sketch "Esboço1" along normal blind 6 contours L405 L407 L583 A22 A27 A28 | L391 L398 L579 A25 bodies 18 19
extrude "Extrusão90" add sketch "Esboço1" along normal blind 2 contours L386 L405 L580 L581 L582 L583 | L405 L407 L582 L583 | L386 L405 L581 L582 | L386 L405 L407 L582 | L386 L407 L582 L583 | L386 L387 L581 L582 | L386 L407 L582 | L386 L387 L388 L396 L583 | L386 L387 L582 L583 | L386 L387 L580 L581 | L386 L387 L389 L395 L580 | L391 L398 L578 L579 | L391 L409 L576 L577 L578 L579 | L387 L388 L583 | L387 L388 L582 L583 | L387 L395 L580 L581 | L387 L395 L580 | L391 L398 L409 L578 | L391 L409 L577 L578 | L398 L409 L578 L579 | L387 L388 L395 L408 L577 L578 L581 L582 | L388 L396 L582 L583 | L396 L578 L579 L582 L583 | L389 L576 L577 L580 L581 | L389 L395 L580 L581 | L408 L409 L577 L578 | L398 L409 L578 | L389 L395 L408 L409 L576 | L408 L409 L576 L577 | L408 L409 L578 L579 | L388 L396 L408 L409 L579 | L389 L395 L577 L581 | L388 L396 L578 L582 | L396 L578 L582 | L389 L577 L581 | L395 L408 L576 | L395 L408 L576 L577 | L388 L408 L578 L579 | L388 L408 L579 | L389 L395 L576 L577 | L388 L396 L578 L579 bodies 18
extrude "Extrusão91" add sketch "Esboço1" along normal blind 4 separate body contours A12 L404 L405 A17 A19 A23 A26 A29 A30 S1 L585 | L157 L194 A13 L406 L407 A15 A16 A23 A26 A29 A30 S0 L584 makes body 20 at (103.6056, 67.771, 4) makes body 21 at (72.3896, 37.2893, 4)
extrude "Extrusão92" add sketch "Esboço1" along normal blind 6 contours L405 L407 A23 A26 A29 A30 bodies 20 21
ref_plane "Plano de trabalho2" through (200, 104.1908, 0) normal (-1, 0, 0) x (0, -1, 0)
mirror "Espelhar3" about plane through (200, 104.1908, 0) normal (-1, 0, 0) of bodies 20 makes body 22
copy_body "Copiar e colar corpos5" bodies 1 16 17 6 11 makes body 23 makes body 24 makes body 25 makes body 26 makes body 27
move_body "Mover4" bodies 23 24 25 26 27 to x (1, 0, 0) y (0, 1, 0) z (0, 0, 1) at (400, 0, 0)
named bodies: "Topo 1", "Esquerda 3 Células", "Direita 3 Células", "Esquerda 4 Células", "Direita 4 Células", "Círculo", "Conexão Esquerda", "Conexão Direita", "Topo 2", "Esquerda Baixo 2", "Direita Baixo 2", "Esquerda Meio 2", "Direita Meio 2"
